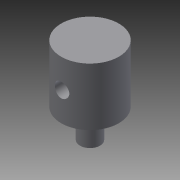
# Autodesk Inventor part: right angle rod holder
Saved by Autodesk Inventor 2014 SP1 (Build 180222100, 222)
## iProperties
Created: 2014-01-31
Part Number: right angle rod holder
Material: Generic
Document SubType Name: Modeling
Designer: Michael
Density: 1 g/cm^3
Appearance: Default
Mass: 12.8588 g
Surface Area: 38.2898 cm^2
Volume: 12.8588 cm^3
Author: Michael
Autodesk Inventor part; units mm, degrees
ref_plane "YZ Plane" through (0, 0, 0) normal (1, 0, 0) x (0, 1, 0)
ref_plane "XZ Plane" through (0, 0, 0) normal (0, 1, 0) x (-1, 0, 0)
ref_plane "XY Plane" through (0, 0, 0) normal (0, 0, 1) x (1, 0, 0)
sketch "Sketch1" plane through (0, 0, 0) normal (0, 0, 1) x (1, 0, 0)
  line L0 (0, 0) -> (0, 38.1)
  line L1 (0, 38.1) -> (12.7, 38.1)
  line L2 (12.7, 38.1) -> (12.7, 12.7)
  line L3 (12.7, 12.7) -> (4.445, 12.7)
  line L4 (4.445, 12.7) -> (4.445, 0)
  line L5 (4.445, 0) -> (0, 0)
  dimension "d0" = 38.1
  dimension "d1" = 12.7
  dimension "d2" = 25.4
  dimension "d3" = 8.255
  constraints: 12 end point, 4 perpendicular, 1 parallel, 1 vertical
  measures "d0" distance of L0.start L0.end
  measures "d1" distance of L0.end L1.end
  measures "d2" distance of L1.end L2.end
  measures "d3" distance of L2.end L3.end
revolve "Revolution1" add sketch "Sketch1" angle 360 about axis through (0, 0, 0) along (0, 1, 0)
sketch "Sketch2" plane through (0, 0, 0) normal (0, 0, 1) x (1, 0, 0)
  line L0 (-12.7, 38.1) -> (12.7, 38.1) projected
  line L1 (12.7, 38.1) -> (12.7, 12.7) projected
  line L2 (12.7, 12.7) -> (4.445, 12.7) projected
  line L3 (4.445, 12.7) -> (4.445, 0) projected
  line L4 (4.445, 0) -> (-4.445, 0) projected
  line L5 (-4.445, 0) -> (-4.445, 12.7) projected
  line L6 (-4.445, 12.7) -> (-12.7, 12.7) projected
  line L7 (-12.7, 12.7) -> (-12.7, 38.1) projected
  circle A0 centre (0, 25.4) radius 3.175
  point P0 (0, 0)
  dimension "d5" = 6.35
  constraints: 1 centre point
  measures "d5" diameter of A0
extrude "Extrusion1" cut sketch "Sketch2" along normal through all both and the other way through all contours A0
body "Solid1"
